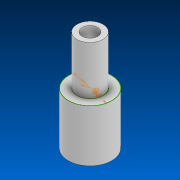
# Autodesk Inventor part: Motor Belt Tensioner Inside
Saved by Autodesk Inventor 2022 (Build 260153000, 153)
## iProperties
Created: 2022-04-08
Part Number: Motor Belt Tensioner Inside
Material: Generic
Document SubType Name: Modeling
Designer: score_nygvs6w
Density: 1 g/cm^3
Appearance: Default
Author: score_nygvs6w
Autodesk Inventor part; units mm, degrees
ref_plane "YZ Plane" through (0, 0, 0) normal (1, 0, 0) x (0, 1, 0)
ref_plane "XZ Plane" through (0, 0, 0) normal (0, 1, 0) x (-1, 0, 0)
ref_plane "XY Plane" through (0, 0, 0) normal (0, 0, 1) x (1, 0, 0)
sketch "Sketch1" plane through (0, 0, 0) normal (0, 1, 0) x (-1, 0, 0)
  circle A0 centre (0, 0) radius 3.81
  circle A1 centre (0, 0) radius 2.286
  circle A2 centre (0, 0) radius 6.35
  dimension "d0" = 7.62
  dimension "d1" = 4.572
  dimension "d2" = 12.7
  constraints: 3 centre point, 3 coincident
  measures "d0" diameter of A0
  measures "d1" diameter of A1
  measures "d2" diameter of A2
extrude "Extrusion1" add sketch "Sketch1" against normal blind 15.24 contours A0 | A2
extrude "Extrusion2" add sketch "Sketch1" along normal blind 14.224 contours A0
body "Solid1"
